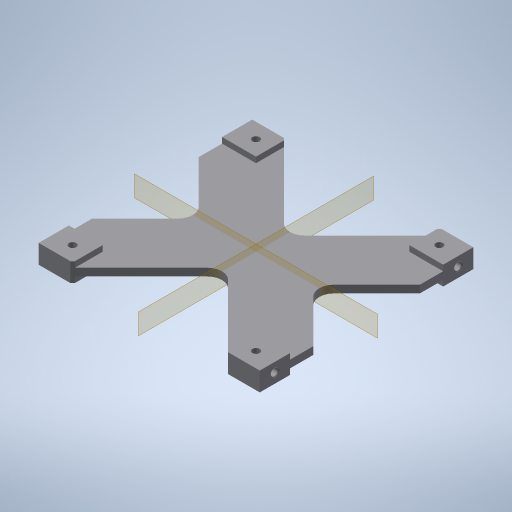
# Autodesk Inventor part: RT-IHU_heatsink
Saved by Autodesk Inventor 2023 (Build 270158000, 158)
## iProperties
Created: 2019-08-10
Part Number: RT-IHU_heatsink
Material: Generic
Document SubType Name: Modeling
Designer: RDavis
Density: 1 g/cm^3
Appearance: Default
Author: RDavis
Autodesk Inventor part; units mm, degrees
ref_plane "YZ Plane" through (0, 0, 0) normal (1, 0, 0) x (0, 1, 0)
ref_plane "XZ Plane" through (0, 0, 0) normal (0, 1, 0) x (-1, 0, 0)
ref_plane "XY Plane" through (0, 0, 0) normal (0, 0, 1) x (1, 0, 0)
sketch "Sketch1" plane through (0, 0, 0) normal (0, 0, 1) x (1, 0, 0)
  circle A0 centre (-39.5, 39.5) radius 1.5875
  circle A1 centre (39.5, 39.5) radius 1.5875
  circle A2 centre (39.5, -39.5) radius 1.5875
  circle A3 centre (-39.5, -39.5) radius 1.5875
  line L0 (0, 0) -> (0, 46)
  line L1 (0, 0) -> (49.2895, 0)
  line L2 (-4.4901, 16.5099) -> (-33.9803, 46)
  line L3 (4.4901, 16.5099) -> (33.9803, 46)
  line L4 (-33.9803, -46) -> (-4.4901, -16.5099)
  line L5 (4.4901, -16.5099) -> (33.9803, -46)
  line L6 (-47.625, 46) -> (-33.9803, 46)
  line L7 (33.9803, 46) -> (47.625, 46)
  line L8 (47.625, -46) -> (33.9803, -46)
  line L9 (-33.9803, -46) -> (-47.625, -46)
  arc A4 (-4.4901, 16.5099) -> (4.4901, 16.5099) centre (0, 21) ccw
  arc A5 (4.4901, -16.5099) -> (-4.4901, -16.5099) centre (0, -21) ccw
  line L10 (-47.625, 22.9803) -> (-29.1349, 4.4901)
  line L11 (-29.1349, -4.4901) -> (-47.625, -22.9803)
  line L12 (47.625, 22.9803) -> (29.1349, 4.4901)
  line L13 (29.1349, -4.4901) -> (47.625, -22.9803)
  arc A6 (-29.1349, -4.4901) -> (-29.1349, 4.4901) centre (-33.625, 0) ccw
  arc A7 (29.1349, 4.4901) -> (29.1349, -4.4901) centre (33.625, 0) ccw
  line L14 (47.625, 46) -> (47.625, 22.9803)
  line L15 (47.625, -22.9803) -> (47.625, -46)
  line L16 (-47.625, -46) -> (-47.625, -22.9803)
  line L17 (-47.625, 22.9803) -> (-47.625, 46)
  point P0 (0, 12.0197)
  point P1 (0, -12.0197)
  point P2 (-24.6447, 0)
  point P3 (24.6447, 0)
  dimension "d0" = 79
  dimension "d1" = 79
  dimension "d2" = 3.175
  dimension "d5" = 6.35
  dimension "d6" = 25
  dimension "d7" = 25
  dimension "d8" = 92
  dimension "d9" = 6.35
  dimension "d10" = 95.25
  dimension "d11" = 14
  constraints: 36 end point, 12 perpendicular, 9 parallel, 9 point on line, 8 centre point, 8 point on circle, 8 tangent, 5 equal radius, 4 collinear, 3 horizontal, 3 symmetric about line, 1 horizontal alignment, 1 midpoint, 1 vertical, 1 vertical alignment, 2 other
  measures "d0" distance of A2.centre A1.centre
  measures "d1" distance of A1.centre A0.centre
  measures "d2" diameter of A0
  measures "d5" radius of A4
  measures "d6" distance from line of L7 A4.centre
  measures "d7" distance from line of A5.centre L8
  measures "d8" distance between parallel lines of L8 L7
  measures "d9" radius of A6
  measures "d10" distance between parallel lines of L14 L17
  measures "d11" distance from line of L16 A6.centre
extrude "Extrusion1" add sketch "Sketch1" along normal mid plane 8.15
sketch "Sketch2" plane through (0, 0, 4.075) normal (0, 0, 1) x (1, 0, 0)
  circle A0 centre (-39.5, -39.5) radius 1.5875 projected
  circle A1 centre (39.5, 39.5) radius 1.5875 projected
  circle A2 centre (-39.5, 39.5) radius 1.5875 projected
  line L0 (-33.9803, 46) -> (-47.625, 46) projected
  line L1 (-47.625, 46) -> (-47.625, 22.9803) projected
  line L2 (-47.625, -46) -> (-33.9803, -46) projected
  line L3 (47.625, 46) -> (33.9803, 46) projected
  line L4 (-33, 46) -> (-33, 33)
  line L5 (-33, 33) -> (-47.625, 33)
  line L6 (-47.625, 33) -> (-47.625, -33)
  line L7 (-47.625, -33) -> (-33, -33)
  line L8 (-33, -33) -> (-33, -46)
  line L9 (-33, -46) -> (33, -46)
  line L10 (33, -46) -> (33, -33)
  line L11 (33, -33) -> (47.625, -33)
  line L12 (47.625, -33) -> (47.625, 33)
  line L13 (47.625, 33) -> (33, 33)
  line L14 (33, 33) -> (33, 46)
  line L15 (33, 46) -> (-33, 46)
  point P0 (0, 0)
  dimension "d14" = 6.5
  dimension "d15" = 6.5
  dimension "d16" = 6.5
  dimension "d17" = 6.5
  constraints: 24 end point, 5 collinear, 4 parallel, 3 equal length, 3 horizontal, 3 perpendicular, 2 vertical
  measures "d14" distance from line of A2.centre L5
  measures "d15" distance from line of A2.centre L4
  measures "d16" distance from line of A1.centre L14
  measures "d17" distance from line of A0.centre L7
extrude "Extrusion2" cut sketch "Sketch2" against normal blind 2.45 contours L5 L4 L15 L14 L13 L12 L11 L10 L9 L8 L7 L6 L1
mirror "Mirror1" about plane through (0, 0, 0) normal (0, 0, 1) of "Extrusion2"
hole "Hole1" at (47.625, 39.5, 0) direction (-1, 0, 0) diameter 3.048 depth 5.3848 tip angle 118 countersink diameter 3.937 countersink angle 120
mirror "Mirror2" about plane through (0, 0, 0) normal (0, 1, 0) of "Hole1"
mirror "Mirror3" about plane through (0, 0, 0) normal (1, 0, 0) of "Hole1", "Mirror2"
ref_plane "Work Plane3" through (-27.275, 0, 1.625) normal (0, -1, 0) x (1, 0, 0)
ref_plane "Work Plane4" through (0, -14.65, 1.625) normal (1, 0, 0) x (0, 0, -1)
body "Solid1"
